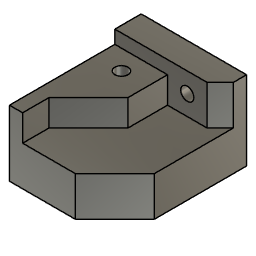
TAsk1Doneee v1 (Autodesk Fusion 360 design; units mm, degrees)
Autodesk Fusion 360 part; units mm, degrees
note: some values were not read from the file. Chosen so that the rebuilt part matches the saved one: a direction.
sketch "Sketch1" plane through (0, 0, 0) normal (0, 0, 1) x (1, 0, 0)
  line L0 (-28.1365, 21.3293) -> (-12.1365, 21.3293)
  line L1 (-12.1365, 21.3293) -> (-12.1365, 1.3293)
  line L2 (-12.1365, 1.3293) -> (-28.1365, 1.3293)
  line L3 (-28.1365, 1.3293) -> (-28.1365, 21.3293)
  dimension "d1" = 16
  dimension "d2" = 20
  constraint horizontal L0
  constraint vertical L1
  constraint horizontal L2
  constraint vertical L3
  measures "d1" distance of L0.start L0.end
  measures "d2" distance of L0.start L2.end
extrude "Extrude1" add sketch "Sketch1" along normal blind 6
chamfer "Chamfer1" distance 6 angle 45 1 edges at (-12.1365, 1.3293, 3)
sketch "Sketch2" plane through (0, 0, 6) normal (0, 0, 1) x (-1, 0, 0)
  line L0 (18.1365, -1.3293) -> (12.1365, -7.3293)
  line L1 (12.1365, -7.3293) -> (12.1365, -21.3293)
  line L2 (12.1365, -21.3293) -> (28.1365, -21.3293)
  line L3 (28.1365, -21.3293) -> (28.1365, -1.3293)
  line L4 (28.1365, -1.3293) -> (18.1365, -1.3293)
  line L5 (28.1365, -21.3293) -> (12.1365, -21.3293)
  line L6 (12.1365, -21.3293) -> (12.1365, -17.3293)
  line L7 (12.1365, -17.3293) -> (28.1365, -17.3293)
  line L8 (28.1365, -17.3293) -> (28.1365, -21.3293)
  dimension "d6" = 16
  dimension "d7" = 4
  constraint horizontal L5
  constraint vertical L6
  constraint horizontal L7
  constraint vertical L8
  constraint coincident L2.end L3.start
  measures "d6" distance of L2.end L1.end
  measures "d7" distance of L2.end L7.end
extrude "Extrude2" add sketch "Sketch2" along normal blind 6 contours L1 L2 L3 L5 L6 L7 L8
chamfer "Chamfer2" distance 2 angle 45 1 edges at (-12.1365, 17.3293, 9)
sketch "Sketch3" plane through (0, 17.3293, 0) normal (0, -1, 0) x (1, 0, 0)
  line L0 (-14.1365, 6) -> (-14.1365, 12)
  line L1 (-14.1365, 12) -> (-28.1365, 12)
  line L2 (-28.1365, 12) -> (-28.1365, 6)
  line L3 (-28.1365, 6) -> (-14.1365, 6)
  line L4 (-28.1365, 6) -> (-20.1365, 6)
  line L5 (-20.1365, 6) -> (-20.1365, 10)
  line L6 (-20.1365, 10) -> (-28.1365, 10)
  line L7 (-28.1365, 10) -> (-28.1365, 6)
  dimension "d11" = 8
  dimension "d12" = 4
  constraint horizontal L4
  constraint vertical L5
  constraint horizontal L6
  constraint vertical L7
  constraint coincident L2.end L3.start
  measures "d11" distance of L2.end L4.end
  measures "d12" distance of L2.end L6.end
extrude "Extrude3" add sketch "Sketch3" along normal blind 6 contours L2 L3 L4 L5 L6 L7
extrude "Extrude4" add 1 faces at (-22.8032, 11.3293, 7.3333) along direction (0, -1, 0) blind 6
chamfer "Chamfer3" distance 6 angle 45 1 edges at (-20.1365, 5.3293, 8)
extrude "Extrude5" add 1 faces at (-26.8032, 5.3293, 7.3333) along direction (0, -1, 0) blind 4
move_body "Move1" bodies 1 to x (1, 0, 0) y (0, 1, 0) z (0, 0, 1) at (0.135, 0, 0)
sketch "Sketch4" plane through (0, 17.3293, 0) normal (0, -1, 0) x (1, 0, 0)
  line L0 (-20.0015, 10) -> (-20.0015, 6)
  line L1 (-20.0015, 6) -> (-14.0015, 6)
  line L2 (-14.0015, 6) -> (-14.0015, 12)
  line L3 (-14.0015, 12) -> (-28.0015, 12)
  line L4 (-28.0015, 12) -> (-28.0015, 10)
  line L5 (-28.0015, 10) -> (-20.0015, 10)
  circle A0 centre (-17, 9) radius 1
  dimension "d20" = 2
  measures "d20" diameter of A0
extrude "Extrude6" cut sketch "Sketch4" against normal through all contours A0
move_body "Move2" bodies 1 to x (1, 0, 0) y (0, 1, 0) z (0, 0, 1) at (0, 1.17, 0)
move_body "Move3" bodies 1 to x (1, 0, 0) y (0, 1, 0) z (0, 0, 1) at (0, 0.5, 0)
sketch "Sketch5" plane through (0, 0, 10) normal (0, 0, 1) x (-1, 0, 0)
  line L0 (26.0015, -6.9993) -> (20.0015, -12.9993)
  line L1 (20.0015, -12.9993) -> (20.0015, -18.9993)
  line L2 (20.0015, -18.9993) -> (28.0015, -18.9993)
  line L3 (28.0015, -18.9993) -> (28.0015, -2.9993)
  line L4 (28.0015, -2.9993) -> (26.0015, -2.9993)
  line L5 (26.0015, -2.9993) -> (26.0015, -6.9993)
  circle A0 centre (30.2556, -17.6884) radius 0.2035
  circle A1 centre (24, -16) radius 1
  dimension "d22" = 2
  measures "d22" diameter of A1
extrude "Extrude7" cut sketch "Sketch5" against normal through all contours A1
